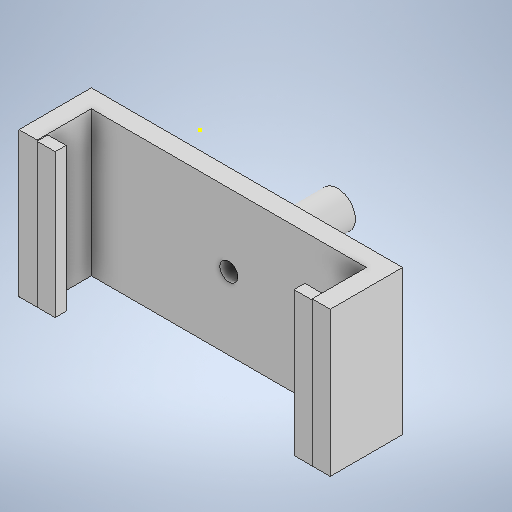
# Autodesk Inventor part: Holder
Saved by Autodesk Inventor 2025 (Build 290162000, 162)
## iProperties
Created: 2025-10-12
Part Number: Holder
Material: Generic
Document SubType Name: Modeling
Designer: parsh
Density: 1 g/cm^3
Appearance: Default
Author: parsh
Autodesk Inventor part; units mm, degrees
ref_plane "YZ Plane" through (0, 0, 0) normal (1, 0, 0) x (0, 1, 0)
ref_plane "XZ Plane" through (0, 0, 0) normal (0, 1, 0) x (-1, 0, 0)
ref_plane "XY Plane" through (0, 0, 0) normal (0, 0, 1) x (1, 0, 0)
sketch "Sketch1" plane through (0, 0, 0) normal (0, 0, 1) x (1, 0, 0)
  circle A0 centre (0, 0) radius 5
  circle A1 centre (0, 0) radius 2.5
  dimension "d0" = 10
  dimension "d1" = 5
  constraints: 2 centre point, 2 coincident
  measures "d0" diameter of A0
  measures "d1" diameter of A1
extrude "Extrusion1" add sketch "Sketch1" along normal blind 25
sketch "Sketch2" plane through (0, 0, 25) normal (0, 0, 1) x (1, 0, 0)
  line L0 (0, 20) -> (38, 20)
  line L1 (38, 20) -> (38, -20)
  line L2 (38, -20) -> (-38, -20)
  line L3 (-38, -20) -> (-38, 20)
  line L4 (-38, 20) -> (0, 20)
  circle A0 centre (0, 0) radius 2.5
  dimension "d4" = 20
  dimension "d6" = 38
  dimension "d7" = 40
  dimension "d8" = 76
  dimension "d9" = 40
  constraints: 10 end point, 2 perpendicular, 1 centre point, 1 coincident, 1 collinear, 1 horizontal, 1 point on line
  measures "d4" distance of point (0, 0) L0.start
  measures "d6" distance of L0.start L0.end
  measures "d7" distance of L0.end L1.end
  measures "d8" distance of L1.end L2.end
  measures "d9" distance of L2.end L3.end
extrude "Extrusion2" add sketch "Sketch2" along normal blind 5
sketch "Sketch3" plane through (0, 0, 30) normal (0, 0, 1) x (1, 0, 0)
  line L0 (38, 20) -> (-38, 20) projected
  line L1 (38, 20) -> (43, 20)
  line L2 (43, 20) -> (43, -20)
  line L3 (43, -20) -> (38, -20)
  line L4 (38, -20) -> (38, 20)
  line L5 (-38, 20) -> (-38, -20) projected
  line L6 (-38, -20) -> (-43, -20)
  line L7 (-43, -20) -> (-43, 20)
  line L8 (-43, 20) -> (-38, 20)
  line L9 (-38, 20) -> (-38, -20)
  point P0 (0, 0)
  dimension "d12" = 5
  dimension "d13" = 40
  dimension "d14" = 5
  constraints: 16 end point, 4 parallel, 2 horizontal, 2 perpendicular
  measures "d12" distance of L2.end L3.end
  measures "d13" distance of L1.end L2.end
  measures "d14" distance of L7.end L8.end
extrude "Extrusion3" add sketch "Sketch3" along normal blind 15 and the other way blind 5
sketch "Sketch4" plane through (-38, -20, 30) normal (1, 0, 0) x (0, 0, -1)
  point P0 (30, 20)
sketch "Sketch5" plane through (-38, -20, 30) normal (1, 0, 0) x (0, 0, -1)
  line L0 (0, 0) -> (-15, 0) projected
  line L1 (-14.9948, 39.7098) -> (-11.9948, 39.7098)
  line L2 (-11.9948, 39.7098) -> (-11.9948, 0)
  line L3 (-11.9948, 0) -> (-14.9948, 0)
  line L4 (-14.9948, 0) -> (-14.9948, 39.7098)
  point P0 (30, 20)
  dimension "d19" = 3
  constraints: 8 end point, 2 parallel, 1 horizontal, 1 perpendicular, 1 point on line
  measures "d19" distance of L2.end L3.end
extrude "Extrusion4" add sketch "Sketch5" along normal blind 5
sketch "Sketch6" plane through (38, -20, 30) normal (-1, 0, 0) x (0, 0, 1)
  line L0 (11.9948, 39.7098) -> (14.9948, 39.7098) projected
  line L1 (11.9948, 39.7098) -> (11.9948, 0) projected
  line L2 (14.9948, 39.7098) -> (11.9948, 39.7098)
  line L3 (11.9948, 39.7098) -> (11.9948, 0)
  line L4 (11.9948, 0) -> (14.9948, 0)
  line L5 (14.9948, 0) -> (14.9948, 39.7098)
  point P0 (-30, 20)
  constraints: 8 end point, 2 parallel, 1 horizontal, 1 perpendicular
extrude "Extrusion5" add sketch "Sketch6" along normal blind 5
body "Solid1"
